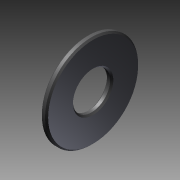
# Autodesk Inventor part: WSSS30-12-2
Saved by Autodesk Inventor 2015 (Build 190159000, 159)
## iProperties
Category: PARTsolutions
Company: MISUMI
Created: 2016-03-29
Part Number: WSSS30-12-2
Catalog Web Link: www.cadenas.de
Description: WSSB, WSSM, WSSS-Metal Washers - Standard Class - T Dimension Selectable -
Vendor: MISUMI
Document SubType Name: Modeling
Designer: psAdmin
Manufacturer: MISUMI
Mass: 1.15454 g
Surface Area: 13.7412 cm^2
Volume: 1.15454 cm^3
Density: 1 g/cm^3
Material: 一般
Appearance: PSOLRGB-175-175-175
PSOL_IDENT_0: {$CADENAS_DATA\23d-libs\misumi\metric\26_washers_collars\wssb.prj},185 {VTYP=3D},{NB=WSSS30-12-2},{L
PSOL_IDENT_1: INA=WSSS30-12-2},{NN=WSSB, WSSM, WSSS},{DATE=10.11.2015 01:59:27},{GEOMDATE=06.10.2015 03:29:00},{VE
PSOL_IDENT_2: RSION=},{LINEID=320},{LINESUBID=-1},{WBVAR=MAT,ST,V,T}  {NB=WSSS30-12-2},{LINA=WSSS30-12-2},{KT=DUMM
PSOL_IDENT_3: Y},{PN=WSSS30-12-2},{TYPE=WSSS},{MAT=304},{ST=-},{STALG= '-','-' },{DALG=4,5,6,8,10,12,13,14,15,16,2
PSOL_IDENT_4: 0,25,30,35,40,50,60},{D=30},{V=12},{VALG=8,10,12,15,16,20,25},{T=2.0},{TALG=1,2,3,4,5,6,8},{C=0.5}
NN: WSSB, WSSM, WSSS
NT: Metal Washers - Standard Class - T Dimension Selectable -
NB: WSSS30-12-2
NBSYN: $PN.
LINA: WSSS30-12-2
PN: WSSS30-12-2
MAT: 304 Stainless Steel
ST: -
D: 30
V: 12
T: 2.0
SUPPLIER: MISUMI
ARTICLENO: WSSS30-12-2
BOMINFO: WSSS30-12-2
CREATOR: CADENAS GmbH
Title: WSSS30-12-2
Author: Cadenas PARTsolutions
Comments: Metal Washers - Standard Class - T Dimension Selectable -
Autodesk Inventor part; units mm, degrees
sketch "Sketch_1" plane through (0, 0, 0) normal (0, 0, 1) x (1, 0, 0)
  line L0 (-3, 0) -> (3, 0)
  line L1 (0, -6.5) -> (0, -14.5)
  line L2 (0, -14.5) -> (0.5, -15)
  line L3 (0.5, -15) -> (1.5, -15)
  line L4 (1.5, -15) -> (2, -14.5)
  line L5 (2, -14.5) -> (2, -6.5)
  line L6 (2, -6.5) -> (1.5, -6)
  line L7 (1.5, -6) -> (0.5, -6)
  line L8 (0.5, -6) -> (0, -6.5)
  constraints: 18 end point
revolve "Revolution1" add sketch "Sketch_1" angle 360 about axis through (-3, 0, 0) along (-1, 0, 0)
ref_plane "a_XY" through (0, 0, 0) normal (1, 0, 0) x (0, 0, -1)
ref_plane "a_YZ" through (0, 0, 0) normal (0, 0, -1) x (0, 1, 0)
ref_plane "a_ZX" through (0, 0, 0) normal (0, 1, 0) x (1, 0, 0)
body "Solid1"
